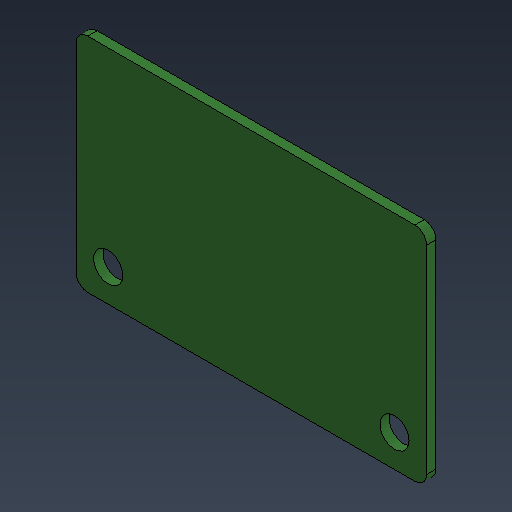
# Autodesk Inventor part: PCB_Main
Saved by Autodesk Inventor 2026.2 (Build 302298010, 298A)
## iProperties
Created: 2026-04-14
Part Number: PCB_Main
Material: Generic
Document SubType Name: Modeling
Designer: szymo
Density: 1 g/cm^3
Appearance: Default(1)
Mass: 0.447459 g
Surface Area: 12.0824 cm^2
Volume: 0.447459 cm^3
Author: szymo
Autodesk Inventor part; units mm, degrees
ref_plane "YZ Plane" through (0, 0, 0) normal (1, 0, 0) x (0, 1, 0)
ref_plane "XZ Plane" through (0, 0, 0) normal (0, 1, 0) x (-1, 0, 0)
ref_plane "XY Plane" through (0, 0, 0) normal (0, 0, 1) x (1, 0, 0)
sketch "Sketch1" plane through (0, 0, 0) normal (0, 0, 1) x (1, 0, 0)
  line L0 (0, 0) -> (30, 0)
  line L1 (30, 0) -> (30, 19)
  line L2 (30, 19) -> (0, 19)
  line L3 (0, 19) -> (0, 0)
  circle A0 centre (2.75, 2.75) radius 2.75
  circle A1 centre (27.25, 2.75) radius 2.75
  circle A2 centre (2.75, 2.75) radius 1.25
  circle A3 centre (27.25, 2.75) radius 1.25
  dimension "d0" = 30
  dimension "d1" = 19
  dimension "d2" = 5.5
  dimension "d3" = 5.5
  dimension "d6" = 2.5
  dimension "d7" = 2.5
  constraints: 8 end point, 4 centre point, 4 tangent, 2 coincident, 2 parallel, 1 horizontal, 1 perpendicular
  measures "d0" distance of L2.end L1.end
  measures "d1" distance of L0.end L1.end
  measures "d2" diameter of A0
  measures "d3" diameter of A1
  measures "d6" diameter of A2
  measures "d7" diameter of A3
extrude "Extrusion1" add sketch "Sketch1" along normal blind 0.8
fillet "Fillet1" radius 1 4 edges at (30, 0, 0.4) (0, 0, 0.4) (0, 19, 0.4) (30, 19, 0.4)
equation "\"d3\" = d2"
body "Solid1"
